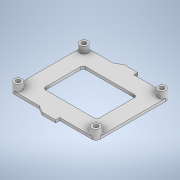
# Autodesk Inventor part: Pi Back Mount
Saved by Autodesk Inventor 2020.3 (Build 243373010, 373A)
## iProperties
Created: 2021-08-29
Part Number: Pi Back Mount
Material: Generic
Document SubType Name: Modeling
Designer: Parker
Density: 1 g/cm^3
Appearance: Default
Author: Parker
Autodesk Inventor part; units mm, degrees
ref_plane "YZ Plane" through (0, 0, 0) normal (1, 0, 0) x (0, 1, 0)
ref_plane "XZ Plane" through (0, 0, 0) normal (0, 1, 0) x (-1, 0, 0)
ref_plane "XY Plane" through (0, 0, 0) normal (0, 0, 1) x (1, 0, 0)
sketch "Sketch1" plane through (0, 0, 0) normal (0, 1, 0) x (-1, 0, 0)
  line L0 (29, 24.5) -> (-29, 24.5) construction
  line L1 (-29, 24.5) -> (-29, -24.5) construction
  line L2 (-29, -24.5) -> (29, -24.5) construction
  line L3 (29, -24.5) -> (29, 24.5) construction
  circle A0 centre (29, 24.5) radius 3
  circle A1 centre (29, -24.5) radius 3
  circle A2 centre (-29, -24.5) radius 3
  circle A3 centre (-29, 24.5) radius 3
  point P0 (0, 0)
  dimension "d0" = 24.5
  dimension "d1" = 29
  dimension "d2" = 58
  dimension "d3" = 49
  dimension "d4" = 6
  dimension "d5" = 6
  dimension "d6" = 6
  dimension "d7" = 6
  constraints: 8 coincident, 8 end point, 4 centre point, 2 parallel, 1 horizontal, 1 perpendicular
  measures "d0" vertical distance of point (0, 0) L0.start
  measures "d1" horizontal distance of point (0, 0) L0.start
  measures "d2" distance of L2.end L1.end
  measures "d3" distance of L1.end L0.end
  measures "d4" diameter of A0
  measures "d5" diameter of A1
  measures "d6" diameter of A2
  measures "d7" diameter of A3
extrude "Extrusion1" add sketch "Sketch1" along normal blind 5
sketch "Sketch2" plane through (-29, 5, 24.5) normal (0, 1, 0) x (1, 0, 0)
  circle A0 centre (0, 0) radius 3 projected
  circle A1 centre (0, 49) radius 3 projected
  circle A2 centre (58, 49) radius 3 projected
  circle A3 centre (58, 0) radius 3 projected
  point P0 (29, 24.5)
hole "Hole1" at (-29, 5, 24.5) at (-29, 5, -24.5) at (29, 5, -24.5) at (29, 5, 24.5) direction (0, -1, 0) diameter 3.3 end through all
sketch "Sketch3" plane through (0, 0, 0) normal (0, 1, 0) x (-1, 0, 0)
  circle A0 centre (29, -24.5) radius 3 projected
  circle A1 centre (29, 24.5) radius 3 projected
  circle A2 centre (-29, 24.5) radius 3 projected
  line L0 (32, -27.5) -> (-32, -27.5)
  line L1 (-32, -27.5) -> (-32, 27.5)
  line L2 (-32, 27.5) -> (32, 27.5)
  line L3 (32, 27.5) -> (32, -27.5)
  circle A3 centre (-29, -24.5) radius 1.65 projected
  circle A4 centre (-29, 24.5) radius 1.65 projected
  circle A5 centre (29, 24.5) radius 1.65 projected
  circle A6 centre (29, -24.5) radius 1.65 projected
  circle A7 centre (-29, -24.5) radius 3 projected
  point P0 (0, 0)
  point P1 (-32, -24.5)
  point P2 (-29, -27.5)
  point P3 (29, -27.5)
  point P4 (32, -24.5)
  point P5 (32, 24.5)
  point P6 (29, 27.5)
  point P7 (-29, 27.5)
  point P8 (-32, 24.5)
  constraints: 8 end point, 2 parallel, 1 horizontal, 1 perpendicular
extrude "Extrusion2" add sketch "Sketch3" against normal blind 2 contours A0 | A0 L0 A7 L1 A2 L2 A1 L3 | A1 | A7 | A2
sketch "Sketch4" plane through (0, 0, 0) normal (0, 1, 0) x (1, 0, 0)
  line L0 (-5, -30.5) -> (5, -30.5)
  line L1 (5, -30.5) -> (5, 30.5)
  line L2 (5, 30.5) -> (-5, 30.5)
  line L3 (-5, 30.5) -> (-5, -30.5)
  line L4 (-5, -30.5) -> (5, 30.5) construction
  line L5 (5, -30.5) -> (-5, 30.5) construction
  line L6 (29, 27.5) -> (-29, 27.5) projected
  arc A0 (-29, -27.5) -> (-32, -24.5) centre (-29, -24.5) ccw projected
  line L7 (-29, -27.5) -> (29, -27.5) projected
  arc A1 (32, -24.5) -> (29, -27.5) centre (29, -24.5) ccw projected
  line L8 (32, -24.5) -> (32, 24.5) projected
  arc A2 (29, 27.5) -> (32, 24.5) centre (29, 24.5) ccw projected
  line L9 (29, 27.5) -> (-29, 27.5) projected
  arc A3 (-32, 24.5) -> (-29, 27.5) centre (-29, 24.5) ccw projected
  line L10 (-32, 24.5) -> (-32, -24.5) projected
  line L11 (-5, -30.5) -> (-10.1962, -27.5)
  line L12 (-5, 30.5) -> (-10.1962, 27.5)
  point P0 (0, 0)
  point P1 (5, 27.5)
  point P2 (5, -27.5)
  dimension "d19" = 10
  dimension "d20" = 3
  dimension "d21" = 6
  dimension "d22" = 6
  constraints: 16 end point, 2 midpoint, 2 parallel, 2 point on line, 1 horizontal, 1 perpendicular
  measures "d19" distance of L2.end L1.end
  measures "d20" distance between parallel lines of L2 L6
  measures "d21" distance of L0.start L11.end
  measures "d22" distance of L2.end L12.end
extrude "Extrusion3" add sketch "Sketch4" against normal up to surface (2 mm away) contours L3 L7 L1 L0 | L11 L7 L3 | L6 L12 L3 | L3 L2 L1 L6
sketch "Sketch5" plane through (0, 0, 0) normal (0, 1, 0) x (1, 0, 0)
  line L0 (20, -15) -> (-20, -15)
  line L1 (-20, -15) -> (-20, 15)
  line L2 (-20, 15) -> (20, 15)
  line L3 (20, 15) -> (20, -15)
  line L4 (20, -15) -> (-20, 15) construction
  line L5 (-20, -15) -> (20, 15) construction
  point P0 (0, 0)
  dimension "d25" = 40
  dimension "d26" = 30
  constraints: 12 end point, 2 midpoint, 2 parallel, 1 horizontal, 1 perpendicular
  measures "d25" distance of L1.end L2.end
  measures "d26" distance of L0.end L1.end
extrude "Extrusion4" cut sketch "Sketch5" against normal through all
fillet "Fillet1" radius 2 4 edges at (-20, -1, 15) (-20, -1, -15) (20, -1, -15) (20, -1, 15)
body "Solid1"
